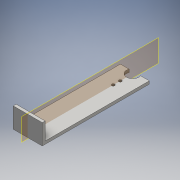
# Autodesk Inventor part: Large Syring Mount
Saved by Autodesk Inventor 2016 (Build 200138000, 138)
## iProperties
Created: 2016-05-08
Part Number: Large Syring Mount
Material: Generic
Document SubType Name: Modeling
Designer: Kenneth Daniel
Density: 1 g/cm^3
Appearance: Default
Author: Kenneth Daniel
Autodesk Inventor part; units mm, degrees
ref_plane "YZ Plane" through (0, 0, 0) normal (1, 0, 0) x (0, 1, 0)
ref_plane "XZ Plane" through (0, 0, 0) normal (0, 1, 0) x (-1, 0, 0)
ref_plane "XY Plane" through (0, 0, 0) normal (0, 0, 1) x (1, 0, 0)
sketch "Sketch1" plane through (0, 0, 0) normal (0, 0, 1) x (1, 0, 0)
  line L0 (-25, -110) -> (-25, 110)
  line L1 (-25, 110) -> (25, 110)
  line L2 (25, 110) -> (25, -110)
  line L3 (25, -110) -> (-25, -110)
  line L4 (-25, -110) -> (25, 110) construction
  line L5 (-25, 110) -> (25, -110) construction
  line L6 (-25, -110) -> (-25, -105)
  line L7 (-25, -105) -> (25, -105)
  point P0 (0, 0)
  dimension "d0" = 220
  dimension "d1" = 50
  dimension "d2" = 5
  constraints: 16 end point, 2 midpoint, 2 parallel, 2 perpendicular, 2 point on line, 1 vertical
  measures "d0" distance of L0.start L0.end
  measures "d1" distance of L0.end L1.end
  measures "d2" distance of L0.start L6.end
extrude "Extrusion1" add sketch "Sketch1" along normal blind 5 contours L0 L1 L2 L7
sketch "Sketch2" plane through (0, 0, 5) normal (0, 0, 1) x (1, 0, 0)
  line L0 (-25, 110) -> (-25, -105) projected
  line L1 (-25, -105) -> (-25, -100)
  line L2 (-25, -100) -> (25, -100)
  line L3 (25, -105) -> (25, 110) projected
  line L4 (25, -100) -> (25, -105)
  line L5 (-25, -105) -> (25, -105) projected
  line L6 (-25, -105) -> (25, -105)
  point P0 (0, 0)
  dimension "d5" = 5
  constraints: 8 end point, 2 perpendicular, 2 point on line, 1 vertical
  measures "d5" distance of L0.end L1.end
extrude "Extrusion2" add sketch "Sketch2" along normal blind 30
sketch "Sketch3" plane through (0, 0, 5) normal (0, 0, 1) x (1, 0, 0)
  line L0 (25, 110) -> (-25, 110) projected
  line L1 (0, 110) -> (-5, 110)
  line L2 (-5, 110) -> (5, 110)
  arc A0 (-5, 110) -> (5, 110) centre (0, 110) ccw
  point P0 (0, 0)
  dimension "d8" = 5
  dimension "d9" = 10
  dimension "d10" = 5
  constraints: 4 end point, 2 point on circle, 2 point on line, 1 centre point, 1 midpoint
  measures "d8" distance of L1.start L1.end
  measures "d9" distance of L1.end L2.end
  measures "d10" radius of A0
extrude "Extrusion3" cut sketch "Sketch3" against normal blind 30
ref_plane "Work Plane1" through (0, -105, 0) normal (1, 0, 0) x (0, 0, -1)
sketch "Sketch4" plane through (25, 110, 5) normal (0, 1, 0) x (1, 0, 0)
  line L0 (0, 0) -> (0, -30) projected
  line L1 (-50, 5) -> (-50, -30) projected
  line L2 (0, 0) -> (-50, 0)
  line L3 (-50, 0) -> (-50, 5)
  line L4 (-50, 5) -> (0, 5)
  line L5 (0, 5) -> (0, 0)
  point P0 (-25, 5)
  constraints: 8 end point, 2 parallel, 1 horizontal, 1 perpendicular
extrude "Extrusion4" cut sketch "Sketch4" against normal blind 30
sketch "Sketch5" plane through (0, 0, 5) normal (0, 0, 1) x (1, 0, 0)
  line L0 (-25, 80) -> (25, 80) projected
  line L1 (0, 80) -> (-10, 80)
  line L2 (-10, 80) -> (10, 80)
  arc A0 (-10, 80) -> (10, 80) centre (0, 80) ccw
  point P0 (0, 0)
  dimension "d15" = 10
  dimension "d16" = 20
  dimension "d17" = 10
  constraints: 4 end point, 2 point on circle, 2 point on line, 1 centre point, 1 midpoint
  measures "d15" distance of L1.start L1.end
  measures "d16" distance of L1.end L2.end
  measures "d17" radius of A0
extrude "Extrusion5" cut sketch "Sketch5" against normal blind 30
sketch "Sketch6" plane through (0, 0, 5) normal (0, 0, 1) x (1, 0, 0)
  line L0 (0, 80) -> (0, 54.77)
  line L1 (0, 54.77) -> (0, 42.6)
  circle A0 centre (0, 54.77) radius 2.5
  circle A1 centre (0, 42.6) radius 2.5
  point P0 (0, 0)
  dimension "d20" = 25.23
  dimension "d21" = 12.17
  dimension "d22" = 5
  dimension "d23" = 5
  constraints: 4 end point, 2 centre point, 2 coincident, 2 vertical
  measures "d20" distance of L0.start L0.end
  measures "d21" distance of L0.end L1.end
  measures "d22" diameter of A0
  measures "d23" diameter of A1
extrude "Extrusion6" cut sketch "Sketch6" against normal blind 30
sketch "Sketch7" plane through (0, 0, 5) normal (0, 0, 1) x (1, 0, 0)
  arc A0 (-10, 80) -> (10, 80) centre (0, 80) ccw projected
  line L0 (10, 80) -> (25, 80) projected
  arc A1 (-10, 80) -> (10, 80) centre (0, 76.3471) ccw
  point P0 (0, 0)
  constraints: 2 point on circle, 1 centre point
extrude "Extrusion7" cut sketch "Sketch7" against normal blind 30
body "Solid1"
